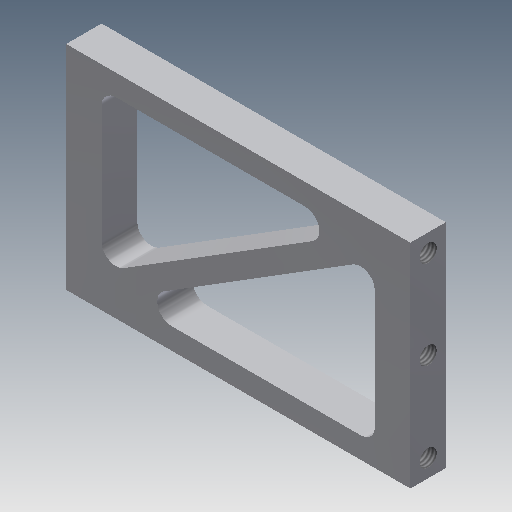
# Autodesk Inventor part: リンク_ふともも_サブフレーム_1_2(予備案)
Saved by Autodesk Inventor 2017.3 (Build 213256000, 256)
## iProperties
Created: 2016-06-03
Part Number: リンク_ふともも_サブフレーム_1_2(予備案)
Material: アルミニウム 2014-T4
Document SubType Name: Modeling
Designer: hiroaki
Density: 2.8 g/cm^3
Appearance: サテン
Author: hiroaki
Autodesk Inventor part; units mm, degrees
ref_plane "YZ Plane" through (0, 0, 0) normal (1, 0, 0) x (0, 1, 0)
ref_plane "XZ Plane" through (0, 0, 0) normal (0, 1, 0) x (-1, 0, 0)
ref_plane "XY Plane" through (0, 0, 0) normal (0, 0, 1) x (1, 0, 0)
sketch "スケッチ1" plane through (0, 0, 0) normal (0, 0, 1) x (1, 0, 0)
  line L0 (-24.25, 15) -> (24.25, 15)
  line L1 (24.25, 15) -> (24.25, -15)
  line L2 (24.25, -15) -> (-24.25, -15)
  line L3 (-24.25, -15) -> (-24.25, 15)
  line L4 (-19.25, 12) -> (19.25, 12) construction
  line L5 (19.25, 12) -> (19.25, -12) construction
  line L6 (19.25, -12) -> (-19.25, -12) construction
  line L7 (-19.25, -12) -> (-19.25, 12) construction
  line L8 (19.25, 12) -> (-19.25, -12) construction
  line L9 (-19.25, -10.2324) -> (-19.25, 12)
  line L10 (-19.25, 12) -> (16.4145, 12)
  line L11 (16.4145, 12) -> (-19.25, -10.2324)
  line L12 (-16.4145, -12) -> (19.25, -12)
  line L13 (19.25, -12) -> (19.25, 10.2324)
  line L14 (19.25, 10.2324) -> (-16.4145, -12)
  line L15 (-24.25, 12.5) -> (24.25, 12.5) construction
  line L16 (24.25, -12.5) -> (-24.25, -12.5) construction
  line L17 (24.25, 12.5) -> (24.25, -12.5) construction
  point P0 (0, 0)
  point P1 (0, 12)
  point P2 (0, 15)
  point P3 (19.25, 0)
  point P4 (24.25, 0)
  dimension "d0" = 5
  dimension "d1" = 3
  dimension "d2" = 1.5
  dimension "d3" = 25
  dimension "d4" = 2.5
  dimension "d16" = 48.5
  constraints: 36 end point, 6 parallel, 5 collinear, 5 horizontal, 5 midpoint, 4 perpendicular, 4 point on line, 2 horizontal alignment, 2 vertical alignment, 1 vertical, 1 other
  measures "d0" distance between parallel lines of L3 L7
  measures "d1" distance between parallel lines of L0 L4
  measures "d2" distance between parallel lines of L8 L11
  measures "d3" distance between parallel lines of L16 L15
  measures "d4" distance between parallel lines of L2 L16
  measures "d16" distance of L0.start L0.end
extrude "押し出し1" add sketch "スケッチ1" along normal blind 5
sketch "スケッチ2" plane through (24.25, -15, 0) normal (1, 0, 0) x (0, 0, -1)
  line L0 (0, 30) -> (-5, 30) projected
  line L1 (-5, 0) -> (-5, 30) projected
  line L2 (0, 15) -> (-5, 15) construction
  point P0 (-2.5, 2.5)
  point P1 (-2.5, 15)
  point P2 (-2.5, 27.5)
  point P3 (-2.5, 30)
  dimension "d7" = 25
  constraints: 3 midpoint, 3 vertical alignment, 2 end point, 1 symmetric about line
  measures "d7" distance of point (-2.5, 27.5) point (-2.5, 2.5)
hole "穴1" at (24.25, -12.5, 2.5) at (24.25, 0, 2.5) at (24.25, 12.5, 2.5) direction (-1, 0, 0) diameter 2.459 depth 3 thread size "M3x0.5" class "6H" standard "ISO Metric profile"
mirror "ミラー1" about plane through (0, 0, 0) normal (1, 0, 0) of "穴1"
fillet "フィレット1" radius 2 6 edges at (-16.4145, -12, 2.5) (-19.25, -10.2324, 2.5) (19.25, 10.2324, 2.5) (19.25, -12, 2.5) (-19.25, 12, 2.5) (16.4145, 12, 2.5)
equation "\"d3\" = d5_1"
equation "\"d7\" = d3"
equation "\"d5_1\" = 25"
